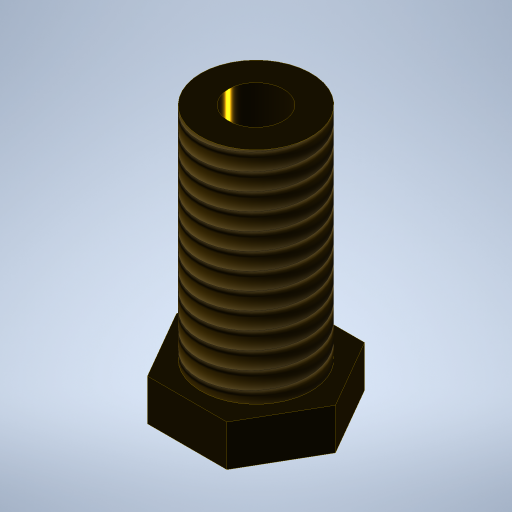
# Autodesk Inventor part: HUDSON-1-87
Saved by Autodesk Inventor 2024.2 (Build 282272000, 272)
## iProperties
Created: 2024-10-05
Part Number: HUDSON-1-87
Material: Generic
Document SubType Name: Modeling
Designer: melim
Density: 1 g/cm^3
Appearance: Metal 2400F Hot
Author: melim
Autodesk Inventor part; units mm, degrees
ref_plane "YZ Plane" through (0, 0, 0) normal (1, 0, 0) x (0, 1, 0)
ref_plane "XZ Plane" through (0, 0, 0) normal (0, 1, 0) x (-1, 0, 0)
ref_plane "XY Plane" through (0, 0, 0) normal (0, 0, 1) x (1, 0, 0)
sketch "Sketch1" plane through (0, 0, 0) normal (0, 1, 0) x (-1, 0, 0)
  line L0 (0, 0) -> (-11.547, 0)
  line L1 (-11.547, 0) -> (-8.6603, 5)
  line L2 (-8.6603, 5) -> (-2.8868, 5)
  line L3 (-2.8868, 5) -> (0, 0)
  line L4 (0, 0) -> (-2.8868, -5)
  line L5 (-2.8868, -5) -> (-8.6603, -5)
  line L6 (-8.6603, -5) -> (-11.547, 0)
  circle A0 centre (-5.7735, 0) radius 4
  circle A1 centre (-5.7735, 0) radius 2
  dimension "d0" = 10
  dimension "d1" = 8
  dimension "d2" = 4
  constraints: 14 end point, 2 centre point, 2 coincident, 1 horizontal, 1 midpoint, 13 other
  measures "d0" distance between parallel lines of L3 L6
  measures "d1" diameter of A0
  measures "d2" diameter of A1
extrude "Extrusion1" add sketch "Sketch1" against normal blind 3
extrude "Extrusion2" add sketch "Sketch1" along normal blind 16 contours A0 L0 A1 | L0 A1 A0
thread "Thread1" size "M8x1.25" class "6g" standard "ANSI Metric M Profile" full length
body "Solid1"
